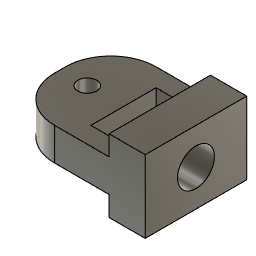
link_2 (Autodesk Fusion 360 design; units mm, degrees)
Autodesk Fusion 360 part; units mm, degrees
sketch "Sketch1" plane through (0, 0, 0) normal (0, 1, 0) x (1, 0, 0)
  line L0 (0, 0) -> (15, 0)
  line L1 (15, 0) -> (15, -9)
  line L2 (15, -9) -> (0, -9)
  line L3 (0, -9) -> (0, 0)
  line L4 (15, -9) -> (17.5, -9)
  line L5 (17.5, 0) -> (15, 0)
  line L6 (17.5, -9) -> (17.5, 0)
  line L7 (17.5, -9) -> (27.5, -9)
  line L8 (27.5, -9) -> (27.5, -14.5)
  line L9 (27.5, -14.5) -> (37.5, -14.5)
  line L10 (37.5, -14.5) -> (37.5, 5.5)
  line L11 (37.5, 5.5) -> (27.5, 5.5)
  line L12 (27.5, 5.5) -> (27.5, 0)
  line L13 (27.5, 0) -> (17.5, 0)
  line L14 (27.5, -9) -> (27.5, 0)
  dimension "d1" = 15
  dimension "d2" = 9
  dimension "d3" = 15
  dimension "d55" = 10
  dimension "d56" = 5.5
  dimension "d57" = 10
  dimension "d58" = 20
  constraint coincident L0.start L3.end
  constraint horizontal L0
  constraint perpendicular L0 L1
  constraint perpendicular L1 L2
  constraint perpendicular L1 L4
  constraint perpendicular L5 L6
  constraint perpendicular L6 L7
  constraint perpendicular L5 L8
  constraint perpendicular L6 L9
  constraint perpendicular L9 L10
  constraint perpendicular L8 L11
  constraint perpendicular L5 L12
  constraint perpendicular L6 L13
  constraint perpendicular L13 L14
  measures "d1" distance of L0.start L0.end
  measures "d2" distance of L0.end L1.end
  measures "d3" distance of L1.end L2.end
  measures "d55" distance of L4.end L7.end
  measures "d56" distance of L7.end L8.end
  measures "d57" distance of L8.end L9.end
  measures "d58" distance of L9.end L10.end
extrude "Extrude2" add sketch "Sketch1" along normal mid plane 28 contours L0 L1 L2 L3 | L1 L4 L5 L6
fillet "Fillet1" radius 12.5 2 edges at (0, -14, 4.5) (0, 14, 4.5)
sketch "Sketch2" plane through (0, 0, 9) normal (0, 0, 1) x (-1, 0, 0)
  line L0 (-12.5, 14) -> (-17.5, 14)
  line L1 (-17.5, -14) -> (-12.5, -14)
  line L2 (0, 0) -> (-7.5, 0) construction
  circle A0 centre (-7.5, 0) radius 2.6
  arc A1 (-12.5, -14) -> (0, -1.5) centre (-12.5, -1.5) ccw
  line L3 (-17.5, 14) -> (-17.5, -14)
  line L4 (0, -1.5) -> (0, 1.5)
  arc A2 (0, 1.5) -> (-12.5, 14) centre (-12.5, 1.5) ccw
  dimension "d28" = 7.5
  dimension "d29" = 5.2
  constraint coincident L2.start origin
  constraint horizontal L2
  constraint coincident L2.end A0.centre
  measures "d28" distance of L2.start L2.end
  measures "d29" diameter of A0
extrude "Extrude4" cut sketch "Sketch2" against normal through all contours A0
extrude "Extrude9" add sketch "Sketch1" against normal blind 5 from surface at 14 contours L6 L7 L13 L14
extrude "Extrude10" add sketch "Sketch1" along normal blind 5 from surface at -14 contours L6 L7 L13 L14
extrude "Extrude11" add sketch "Sketch1" along normal mid plane 28 contours L8 L9 L10 L11 L12 L14
sketch "Sketch4" plane through (37.5, 0, 0) normal (1, 0, 0) x (0, 1, 0)
  line L0 (-14, -5.5) -> (14, -5.5)
  line L1 (14, -5.5) -> (14, 14.5)
  line L2 (14, 14.5) -> (-14, 14.5)
  line L3 (-14, 14.5) -> (-14, -5.5)
  line L4 (0, 14.5) -> (0, 4.5) construction
  line L5 (0, 4.5) -> (-14, 4.5) construction
  circle A0 centre (0, 4.5) radius 5.1
  dimension "d67" = 10
  dimension "d68" = 10.2
  constraint midpoint L2 L4.start
  constraint perpendicular L0 L4
  constraint midpoint L3 L5.end
  constraint coincident L4.end L5.start
  measures "d67" distance of L4.start L4.end
  measures "d68" diameter of A0
extrude "Extrude12" cut sketch "Sketch4" against normal blind 10 contours A0
equation "d27 = ( 25 / 2 ) * 1 mm"
equation "d56 = ( ( 20 - 9 ) / 2 ) * 1 mm"
equation "d59 = ( 28 / 2 ) * 1 mm"
equation "d62 = ( -28 / 2 ) * 1 mm"
equation "d67 = ( 20 / 2 ) * 1 mm"
